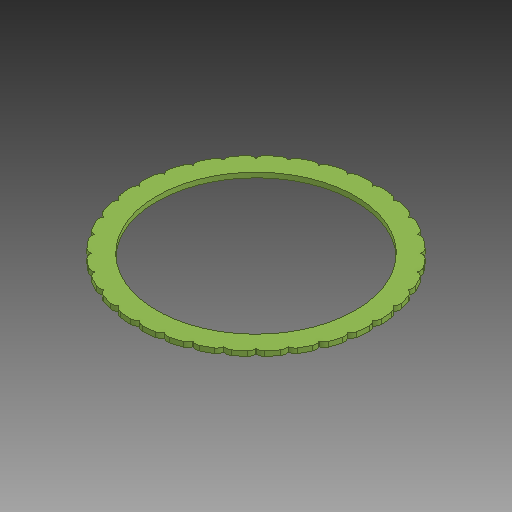
# Autodesk Inventor part: tsop_board
Saved by Autodesk Inventor 2020 (Build 240168000, 168)
## iProperties
Created: 2024-11-04
Part Number: tsop_board
Material: Медь
Document SubType Name: Modeling
Designer: Ivan
Density: 8.94 g/cm^3
Appearance: Оливково-зеленый
Mass: 41.749 g
Surface Area: 58.5361 cm^2
Volume: 4.66991 cm^3
Author: Ivan
Autodesk Inventor part; units mm, degrees
ref_plane "YZ Plane" through (0, 0, 0) normal (1, 0, 0) x (0, 1, 0)
ref_plane "XZ Plane" through (0, 0, 0) normal (0, 1, 0) x (-1, 0, 0)
ref_plane "XY Plane" through (0, 0, 0) normal (0, 0, 1) x (1, 0, 0)
sketch "Эскиз1" plane through (0, 0, 0) normal (0, 1, 0) x (-1, 0, 0)
  line L0 (48.1278, 3.6) -> (42.9278, 3.6)
  line L1 (42.9278, 3.6) -> (42.9278, -3.6)
  line L2 (42.9278, -3.6) -> (48.1278, -3.6)
  line L3 (48.1278, -3.6) -> (48.1278, 3.6)
  line L4 (0, 0) -> (42.9278, 0) construction
  circle A0 centre (0, 0) radius 45.67 construction
  line L5 (45.5278, 3.6) -> (45.5278, -3.6) construction
  line L6 (41.4007, 11.9056) -> (42.8053, 4.844)
  line L7 (46.5008, 12.9201) -> (41.4007, 11.9056)
  line L8 (47.9054, 5.8585) -> (46.5008, 12.9201)
  line L9 (42.8053, 4.844) -> (47.9054, 5.8585)
  line L10 (38.2825, 19.7537) -> (41.0378, 13.1018)
  line L11 (43.0867, 21.7437) -> (38.2825, 19.7537)
  line L12 (45.842, 15.0918) -> (43.0867, 21.7437)
  line L13 (41.0378, 13.1018) -> (45.842, 15.0918)
  line L14 (33.6931, 26.8427) -> (37.6933, 20.8561)
  line L15 (38.0168, 29.7317) -> (33.6931, 26.8427)
  line L16 (42.0169, 23.7451) -> (38.0168, 29.7317)
  line L17 (37.6933, 20.8561) -> (42.0169, 23.7451)
  line L18 (27.809, 32.9002) -> (32.9002, 27.809)
  line L19 (31.4859, 36.5771) -> (27.809, 32.9002)
  line L20 (36.5771, 31.4859) -> (31.4859, 36.5771)
  line L21 (32.9002, 27.809) -> (36.5771, 31.4859)
  line L22 (20.8561, 37.6933) -> (26.8427, 33.6931)
  line L23 (23.7451, 42.0169) -> (20.8561, 37.6933)
  line L24 (29.7317, 38.0168) -> (23.7451, 42.0169)
  line L25 (26.8427, 33.6931) -> (29.7317, 38.0168)
  line L26 (13.1018, 41.0378) -> (19.7537, 38.2825)
  line L27 (15.0918, 45.842) -> (13.1018, 41.0378)
  line L28 (21.7437, 43.0867) -> (15.0918, 45.842)
  line L29 (19.7537, 38.2825) -> (21.7437, 43.0867)
  line L30 (4.844, 42.8053) -> (11.9056, 41.4007)
  line L31 (5.8585, 47.9054) -> (4.844, 42.8053)
  line L32 (12.9201, 46.5008) -> (5.8585, 47.9054)
  line L33 (11.9056, 41.4007) -> (12.9201, 46.5008)
  line L34 (-3.6, 42.9278) -> (3.6, 42.9278)
  line L35 (-3.6, 48.1278) -> (-3.6, 42.9278)
  line L36 (3.6, 48.1278) -> (-3.6, 48.1278)
  line L37 (3.6, 42.9278) -> (3.6, 48.1278)
  line L38 (-11.9056, 41.4007) -> (-4.844, 42.8053)
  line L39 (-12.9201, 46.5008) -> (-11.9056, 41.4007)
  line L40 (-5.8585, 47.9054) -> (-12.9201, 46.5008)
  line L41 (-4.844, 42.8053) -> (-5.8585, 47.9054)
  line L42 (-19.7537, 38.2825) -> (-13.1018, 41.0378)
  line L43 (-21.7437, 43.0867) -> (-19.7537, 38.2825)
  line L44 (-15.0918, 45.842) -> (-21.7437, 43.0867)
  line L45 (-13.1018, 41.0378) -> (-15.0918, 45.842)
  line L46 (-26.8427, 33.6931) -> (-20.8561, 37.6933)
  line L47 (-29.7317, 38.0168) -> (-26.8427, 33.6931)
  line L48 (-23.7451, 42.0169) -> (-29.7317, 38.0168)
  line L49 (-20.8561, 37.6933) -> (-23.7451, 42.0169)
  line L50 (-32.9002, 27.809) -> (-27.809, 32.9002)
  line L51 (-36.5771, 31.4859) -> (-32.9002, 27.809)
  line L52 (-31.4859, 36.5771) -> (-36.5771, 31.4859)
  line L53 (-27.809, 32.9002) -> (-31.4859, 36.5771)
  line L54 (-37.6933, 20.8561) -> (-33.6931, 26.8427)
  line L55 (-42.0169, 23.7451) -> (-37.6933, 20.8561)
  line L56 (-38.0168, 29.7317) -> (-42.0169, 23.7451)
  line L57 (-33.6931, 26.8427) -> (-38.0168, 29.7317)
  line L58 (-41.0378, 13.1018) -> (-38.2825, 19.7537)
  line L59 (-45.842, 15.0918) -> (-41.0378, 13.1018)
  line L60 (-43.0867, 21.7437) -> (-45.842, 15.0918)
  line L61 (-38.2825, 19.7537) -> (-43.0867, 21.7437)
  line L62 (-42.8053, 4.844) -> (-41.4007, 11.9056)
  line L63 (-47.9054, 5.8585) -> (-42.8053, 4.844)
  line L64 (-46.5008, 12.9201) -> (-47.9054, 5.8585)
  line L65 (-41.4007, 11.9056) -> (-46.5008, 12.9201)
  line L66 (-42.9278, -3.6) -> (-42.9278, 3.6)
  line L67 (-48.1278, -3.6) -> (-42.9278, -3.6)
  line L68 (-48.1278, 3.6) -> (-48.1278, -3.6)
  line L69 (-42.9278, 3.6) -> (-48.1278, 3.6)
  line L70 (-41.4007, -11.9056) -> (-42.8053, -4.844)
  line L71 (-46.5008, -12.9201) -> (-41.4007, -11.9056)
  line L72 (-47.9054, -5.8585) -> (-46.5008, -12.9201)
  line L73 (-42.8053, -4.844) -> (-47.9054, -5.8585)
  line L74 (-38.2825, -19.7537) -> (-41.0378, -13.1018)
  line L75 (-43.0867, -21.7437) -> (-38.2825, -19.7537)
  line L76 (-45.842, -15.0918) -> (-43.0867, -21.7437)
  line L77 (-41.0378, -13.1018) -> (-45.842, -15.0918)
  line L78 (-33.6931, -26.8427) -> (-37.6933, -20.8561)
  line L79 (-38.0168, -29.7317) -> (-33.6931, -26.8427)
  line L80 (-42.0169, -23.7451) -> (-38.0168, -29.7317)
  line L81 (-37.6933, -20.8561) -> (-42.0169, -23.7451)
  line L82 (-27.809, -32.9002) -> (-32.9002, -27.809)
  line L83 (-31.4859, -36.5771) -> (-27.809, -32.9002)
  line L84 (-36.5771, -31.4859) -> (-31.4859, -36.5771)
  line L85 (-32.9002, -27.809) -> (-36.5771, -31.4859)
  line L86 (-20.8561, -37.6933) -> (-26.8427, -33.6931)
  line L87 (-23.7451, -42.0169) -> (-20.8561, -37.6933)
  line L88 (-29.7317, -38.0168) -> (-23.7451, -42.0169)
  line L89 (-26.8427, -33.6931) -> (-29.7317, -38.0168)
  line L90 (-13.1018, -41.0378) -> (-19.7537, -38.2825)
  line L91 (-15.0918, -45.842) -> (-13.1018, -41.0378)
  line L92 (-21.7437, -43.0867) -> (-15.0918, -45.842)
  line L93 (-19.7537, -38.2825) -> (-21.7437, -43.0867)
  line L94 (-4.844, -42.8053) -> (-11.9056, -41.4007)
  line L95 (-5.8585, -47.9054) -> (-4.844, -42.8053)
  line L96 (-12.9201, -46.5008) -> (-5.8585, -47.9054)
  line L97 (-11.9056, -41.4007) -> (-12.9201, -46.5008)
  line L98 (3.6, -42.9278) -> (-3.6, -42.9278)
  line L99 (3.6, -48.1278) -> (3.6, -42.9278)
  line L100 (-3.6, -48.1278) -> (3.6, -48.1278)
  line L101 (-3.6, -42.9278) -> (-3.6, -48.1278)
  line L102 (11.9056, -41.4007) -> (4.844, -42.8053)
  line L103 (12.9201, -46.5008) -> (11.9056, -41.4007)
  line L104 (5.8585, -47.9054) -> (12.9201, -46.5008)
  line L105 (4.844, -42.8053) -> (5.8585, -47.9054)
  line L106 (19.7537, -38.2825) -> (13.1018, -41.0378)
  line L107 (21.7437, -43.0867) -> (19.7537, -38.2825)
  line L108 (15.0918, -45.842) -> (21.7437, -43.0867)
  line L109 (13.1018, -41.0378) -> (15.0918, -45.842)
  line L110 (26.8427, -33.6931) -> (20.8561, -37.6933)
  line L111 (29.7317, -38.0168) -> (26.8427, -33.6931)
  line L112 (23.7451, -42.0169) -> (29.7317, -38.0168)
  line L113 (20.8561, -37.6933) -> (23.7451, -42.0169)
  line L114 (32.9002, -27.809) -> (27.809, -32.9002)
  line L115 (36.5771, -31.4859) -> (32.9002, -27.809)
  line L116 (31.4859, -36.5771) -> (36.5771, -31.4859)
  line L117 (27.809, -32.9002) -> (31.4859, -36.5771)
  line L118 (37.6933, -20.8561) -> (33.6931, -26.8427)
  line L119 (42.0169, -23.7451) -> (37.6933, -20.8561)
  line L120 (38.0168, -29.7317) -> (42.0169, -23.7451)
  line L121 (33.6931, -26.8427) -> (38.0168, -29.7317)
  line L122 (41.0378, -13.1018) -> (38.2825, -19.7537)
  line L123 (45.842, -15.0918) -> (41.0378, -13.1018)
  line L124 (43.0867, -21.7437) -> (45.842, -15.0918)
  line L125 (38.2825, -19.7537) -> (43.0867, -21.7437)
  line L126 (42.8053, -4.844) -> (41.4007, -11.9056)
  line L127 (47.9054, -5.8585) -> (42.8053, -4.844)
  line L128 (46.5008, -12.9201) -> (47.9054, -5.8585)
  line L129 (41.4007, -11.9056) -> (46.5008, -12.9201)
  line L130 (42.8053, 4.844) -> (42.9278, 3.6) construction
  line L131 (42.9278, 3.6) -> (46.884, 3.9896) construction
  point P0 (45.67, 0)
  point P1 (42.103, 8.3748)
  point P2 (43.9507, 12.4129)
  point P3 (45.3554, 5.3512)
  point P4 (39.6602, 16.4278)
  point P5 (40.6846, 20.7487)
  point P6 (43.4399, 14.0968)
  point P7 (35.6932, 23.8494)
  point P8 (35.855, 28.2872)
  point P9 (39.8551, 22.3006)
  point P10 (30.3546, 30.3546)
  point P11 (29.6475, 34.7386)
  point P12 (34.7386, 29.6475)
  point P13 (23.8494, 35.6932)
  point P14 (22.3006, 39.8551)
  point P15 (28.2872, 35.855)
  point P16 (16.4278, 39.6602)
  point P17 (14.0968, 43.4399)
  point P18 (20.7487, 40.6846)
  point P19 (8.3748, 42.103)
  point P20 (5.3512, 45.3554)
  point P21 (12.4129, 43.9507)
  point P22 (0, 42.9278)
  point P23 (-3.6, 45.5278)
  point P24 (3.6, 45.5278)
  point P25 (-8.3748, 42.103)
  point P26 (-12.4129, 43.9507)
  point P27 (-5.3512, 45.3554)
  point P28 (-16.4278, 39.6602)
  point P29 (-20.7487, 40.6846)
  point P30 (-14.0968, 43.4399)
  point P31 (-23.8494, 35.6932)
  point P32 (-28.2872, 35.855)
  point P33 (-22.3006, 39.8551)
  point P34 (-30.3546, 30.3546)
  point P35 (-34.7386, 29.6475)
  point P36 (-29.6475, 34.7386)
  point P37 (-35.6932, 23.8494)
  point P38 (-39.8551, 22.3006)
  point P39 (-35.855, 28.2872)
  point P40 (-39.6602, 16.4278)
  point P41 (-43.4399, 14.0968)
  point P42 (-40.6846, 20.7487)
  point P43 (-42.103, 8.3748)
  point P44 (-45.3554, 5.3512)
  point P45 (-43.9507, 12.4129)
  point P46 (-42.9278, 0)
  point P47 (-45.5278, -3.6)
  point P48 (-45.5278, 3.6)
  point P49 (-42.103, -8.3748)
  point P50 (-43.9507, -12.4129)
  point P51 (-45.3554, -5.3512)
  point P52 (-39.6602, -16.4278)
  point P53 (-40.6846, -20.7487)
  point P54 (-43.4399, -14.0968)
  point P55 (-35.6932, -23.8494)
  point P56 (-35.855, -28.2872)
  point P57 (-39.8551, -22.3006)
  point P58 (-30.3546, -30.3546)
  point P59 (-29.6475, -34.7386)
  point P60 (-34.7386, -29.6475)
  point P61 (-23.8494, -35.6932)
  point P62 (-22.3006, -39.8551)
  point P63 (-28.2872, -35.855)
  point P64 (-16.4278, -39.6602)
  point P65 (-14.0968, -43.4399)
  point P66 (-20.7487, -40.6846)
  point P67 (-8.3748, -42.103)
  point P68 (-5.3512, -45.3554)
  point P69 (-12.4129, -43.9507)
  point P70 (0, -42.9278)
  point P71 (3.6, -45.5278)
  point P72 (-3.6, -45.5278)
  point P73 (8.3748, -42.103)
  point P74 (12.4129, -43.9507)
  point P75 (5.3512, -45.3554)
  point P76 (16.4278, -39.6602)
  point P77 (20.7487, -40.6846)
  point P78 (14.0968, -43.4399)
  point P79 (23.8494, -35.6932)
  point P80 (28.2872, -35.855)
  point P81 (22.3006, -39.8551)
  point P82 (30.3546, -30.3546)
  point P83 (34.7386, -29.6475)
  point P84 (29.6475, -34.7386)
  point P85 (35.6932, -23.8494)
  point P86 (39.8551, -22.3006)
  point P87 (35.855, -28.2872)
  point P88 (39.6602, -16.4278)
  point P89 (43.4399, -14.0968)
  point P90 (40.6846, -20.7487)
  point P91 (42.103, -8.3748)
  point P92 (45.3554, -5.3512)
  point P93 (43.9507, -12.4129)
sketch "Эскиз3" plane through (0, 0, 0) normal (0, 1, 0) x (-1, 0, 0)
  line L0 (42.8053, 4.844) -> (42.9278, 3.6) construction
  line L1 (42.8666, 4.222) -> (50.4728, 4.9711) construction
  line L2 (48.1278, -3.6) -> (48.1278, 3.6)
  line L3 (48.1278, -0.05) -> (48.1278, 0.05)
  line L4 (48.1278, 2.45) -> (49.3278, 2.45) construction
  arc A0 (48.1278, 0.05) -> (49.3278, 2.45) centre (46.3278, 2.45) ccw
  line L5 (49.3278, 2.45) -> (49.3278, 0) construction
  line L6 (0, 0) -> (42.9278, 0) construction
  arc A1 (49.3278, -2.45) -> (48.1278, -0.05) centre (46.3278, -2.45) ccw
  arc A2 (47.1933, 9.4383) -> (47.9021, 12.0263) centre (44.9597, 11.441) ccw
  arc A3 (48.858, 7.2205) -> (47.2128, 9.3402) centre (45.9156, 6.6352) ccw
  line L7 (47.2128, 9.3402) -> (47.1933, 9.4383)
  arc A4 (44.4452, 18.4639) -> (44.6354, 21.1405) centre (41.8638, 19.9924) ccw
  arc A5 (46.5106, 16.6134) -> (44.4835, 18.3715) centre (43.7389, 15.4654) ccw
  line L8 (44.4835, 18.3715) -> (44.4452, 18.4639)
  arc A6 (39.9891, 26.78) -> (39.6535, 29.4422) centre (37.1591, 27.7755) ccw
  arc A7 (42.3758, 25.368) -> (40.0446, 26.6968) centre (39.8813, 23.7013) ccw
  line L9 (40.0446, 26.6968) -> (39.9891, 26.78)
  arc A8 (33.9962, 34.0669) -> (33.1476, 36.6125) centre (31.0263, 34.4911) ccw
  arc A9 (36.6125, 33.1476) -> (34.0669, 33.9962) centre (34.4911, 31.0263) ccw
  line L10 (34.0669, 33.9962) -> (33.9962, 34.0669)
  arc A10 (26.6968, 40.0446) -> (25.368, 42.3758) centre (23.7013, 39.8813) ccw
  arc A11 (29.4422, 39.6535) -> (26.78, 39.9891) centre (27.7755, 37.1591) ccw
  line L11 (26.78, 39.9891) -> (26.6968, 40.0446)
  arc A12 (18.3715, 44.4835) -> (16.6134, 46.5106) centre (15.4654, 43.7389) ccw
  arc A13 (21.1405, 44.6354) -> (18.4639, 44.4452) centre (19.9924, 41.8638) ccw
  line L12 (18.4639, 44.4452) -> (18.3715, 44.4835)
  arc A14 (9.3402, 47.2128) -> (7.2205, 48.858) centre (6.6352, 45.9156) ccw
  arc A15 (12.0263, 47.9021) -> (9.4383, 47.1933) centre (11.441, 44.9597) ccw
  line L13 (9.4383, 47.1933) -> (9.3402, 47.2128)
  arc A16 (-0.05, 48.1278) -> (-2.45, 49.3278) centre (-2.45, 46.3278) ccw
  arc A17 (2.45, 49.3278) -> (0.05, 48.1278) centre (2.45, 46.3278) ccw
  line L14 (0.05, 48.1278) -> (-0.05, 48.1278)
  arc A18 (-9.4383, 47.1933) -> (-12.0263, 47.9021) centre (-11.441, 44.9597) ccw
  arc A19 (-7.2205, 48.858) -> (-9.3402, 47.2128) centre (-6.6352, 45.9156) ccw
  line L15 (-9.3402, 47.2128) -> (-9.4383, 47.1933)
  arc A20 (-18.4639, 44.4452) -> (-21.1405, 44.6354) centre (-19.9924, 41.8638) ccw
  arc A21 (-16.6134, 46.5106) -> (-18.3715, 44.4835) centre (-15.4654, 43.7389) ccw
  line L16 (-18.3715, 44.4835) -> (-18.4639, 44.4452)
  arc A22 (-26.78, 39.9891) -> (-29.4422, 39.6535) centre (-27.7755, 37.1591) ccw
  arc A23 (-25.368, 42.3758) -> (-26.6968, 40.0446) centre (-23.7013, 39.8813) ccw
  line L17 (-26.6968, 40.0446) -> (-26.78, 39.9891)
  arc A24 (-34.0669, 33.9962) -> (-36.6125, 33.1476) centre (-34.4911, 31.0263) ccw
  arc A25 (-33.1476, 36.6125) -> (-33.9962, 34.0669) centre (-31.0263, 34.4911) ccw
  line L18 (-33.9962, 34.0669) -> (-34.0669, 33.9962)
  arc A26 (-40.0446, 26.6968) -> (-42.3758, 25.368) centre (-39.8813, 23.7013) ccw
  arc A27 (-39.6535, 29.4422) -> (-39.9891, 26.78) centre (-37.1591, 27.7755) ccw
  line L19 (-39.9891, 26.78) -> (-40.0446, 26.6968)
  arc A28 (-44.4835, 18.3715) -> (-46.5106, 16.6134) centre (-43.7389, 15.4654) ccw
  arc A29 (-44.6354, 21.1405) -> (-44.4452, 18.4639) centre (-41.8638, 19.9924) ccw
  line L20 (-44.4452, 18.4639) -> (-44.4835, 18.3715)
  arc A30 (-47.2128, 9.3402) -> (-48.858, 7.2205) centre (-45.9156, 6.6352) ccw
  arc A31 (-47.9021, 12.0263) -> (-47.1933, 9.4383) centre (-44.9597, 11.441) ccw
  line L21 (-47.1933, 9.4383) -> (-47.2128, 9.3402)
  arc A32 (-48.1278, -0.05) -> (-49.3278, -2.45) centre (-46.3278, -2.45) ccw
  arc A33 (-49.3278, 2.45) -> (-48.1278, 0.05) centre (-46.3278, 2.45) ccw
  line L22 (-48.1278, 0.05) -> (-48.1278, -0.05)
  arc A34 (-47.1933, -9.4383) -> (-47.9021, -12.0263) centre (-44.9597, -11.441) ccw
  arc A35 (-48.858, -7.2205) -> (-47.2128, -9.3402) centre (-45.9156, -6.6352) ccw
  line L23 (-47.2128, -9.3402) -> (-47.1933, -9.4383)
  arc A36 (-44.4452, -18.4639) -> (-44.6354, -21.1405) centre (-41.8638, -19.9924) ccw
  arc A37 (-46.5106, -16.6134) -> (-44.4835, -18.3715) centre (-43.7389, -15.4654) ccw
  line L24 (-44.4835, -18.3715) -> (-44.4452, -18.4639)
  arc A38 (-39.9891, -26.78) -> (-39.6535, -29.4422) centre (-37.1591, -27.7755) ccw
  arc A39 (-42.3758, -25.368) -> (-40.0446, -26.6968) centre (-39.8813, -23.7013) ccw
  line L25 (-40.0446, -26.6968) -> (-39.9891, -26.78)
  arc A40 (-33.9962, -34.0669) -> (-33.1476, -36.6125) centre (-31.0263, -34.4911) ccw
  arc A41 (-36.6125, -33.1476) -> (-34.0669, -33.9962) centre (-34.4911, -31.0263) ccw
  line L26 (-34.0669, -33.9962) -> (-33.9962, -34.0669)
  arc A42 (-26.6968, -40.0446) -> (-25.368, -42.3758) centre (-23.7013, -39.8813) ccw
  arc A43 (-29.4422, -39.6535) -> (-26.78, -39.9891) centre (-27.7755, -37.1591) ccw
  line L27 (-26.78, -39.9891) -> (-26.6968, -40.0446)
  arc A44 (-18.3715, -44.4835) -> (-16.6134, -46.5106) centre (-15.4654, -43.7389) ccw
  arc A45 (-21.1405, -44.6354) -> (-18.4639, -44.4452) centre (-19.9924, -41.8638) ccw
  line L28 (-18.4639, -44.4452) -> (-18.3715, -44.4835)
  arc A46 (-9.3402, -47.2128) -> (-7.2205, -48.858) centre (-6.6352, -45.9156) ccw
  arc A47 (-12.0263, -47.9021) -> (-9.4383, -47.1933) centre (-11.441, -44.9597) ccw
  line L29 (-9.4383, -47.1933) -> (-9.3402, -47.2128)
  arc A48 (0.05, -48.1278) -> (2.45, -49.3278) centre (2.45, -46.3278) ccw
  arc A49 (-2.45, -49.3278) -> (-0.05, -48.1278) centre (-2.45, -46.3278) ccw
  line L30 (-0.05, -48.1278) -> (0.05, -48.1278)
  arc A50 (9.4383, -47.1933) -> (12.0263, -47.9021) centre (11.441, -44.9597) ccw
  arc A51 (7.2205, -48.858) -> (9.3402, -47.2128) centre (6.6352, -45.9156) ccw
  line L31 (9.3402, -47.2128) -> (9.4383, -47.1933)
  arc A52 (18.4639, -44.4452) -> (21.1405, -44.6354) centre (19.9924, -41.8638) ccw
  arc A53 (16.6134, -46.5106) -> (18.3715, -44.4835) centre (15.4654, -43.7389) ccw
  line L32 (18.3715, -44.4835) -> (18.4639, -44.4452)
  arc A54 (26.78, -39.9891) -> (29.4422, -39.6535) centre (27.7755, -37.1591) ccw
  arc A55 (25.368, -42.3758) -> (26.6968, -40.0446) centre (23.7013, -39.8813) ccw
  line L33 (26.6968, -40.0446) -> (26.78, -39.9891)
  arc A56 (34.0669, -33.9962) -> (36.6125, -33.1476) centre (34.4911, -31.0263) ccw
  arc A57 (33.1476, -36.6125) -> (33.9962, -34.0669) centre (31.0263, -34.4911) ccw
  line L34 (33.9962, -34.0669) -> (34.0669, -33.9962)
  arc A58 (40.0446, -26.6968) -> (42.3758, -25.368) centre (39.8813, -23.7013) ccw
  arc A59 (39.6535, -29.4422) -> (39.9891, -26.78) centre (37.1591, -27.7755) ccw
  line L35 (39.9891, -26.78) -> (40.0446, -26.6968)
  arc A60 (44.4835, -18.3715) -> (46.5106, -16.6134) centre (43.7389, -15.4654) ccw
  arc A61 (44.6354, -21.1405) -> (44.4452, -18.4639) centre (41.8638, -19.9924) ccw
  line L36 (44.4452, -18.4639) -> (44.4835, -18.3715)
  arc A62 (47.2128, -9.3402) -> (48.858, -7.2205) centre (45.9156, -6.6352) ccw
  arc A63 (47.9021, -12.0263) -> (47.1933, -9.4383) centre (44.9597, -11.441) ccw
  line L37 (47.1933, -9.4383) -> (47.2128, -9.3402)
  arc A64 (49.3278, 2.45) -> (48.858, 7.2205) centre (0, 0) ccw
  arc A65 (47.9021, 12.0263) -> (46.5106, 16.6134) centre (0, 0) ccw
  arc A66 (44.6354, 21.1405) -> (42.3758, 25.368) centre (0, 0) ccw
  arc A67 (39.6535, 29.4422) -> (36.6125, 33.1476) centre (0, 0) ccw
  arc A68 (33.1476, 36.6125) -> (29.4422, 39.6535) centre (0, 0) ccw
  arc A69 (25.368, 42.3758) -> (21.1405, 44.6354) centre (0, 0) ccw
  arc A70 (16.6134, 46.5106) -> (12.0263, 47.9021) centre (0, 0) ccw
  arc A71 (7.2205, 48.858) -> (2.45, 49.3278) centre (0, 0) ccw
  arc A72 (-2.45, 49.3278) -> (-7.2205, 48.858) centre (0, 0) ccw
  arc A73 (-12.0263, 47.9021) -> (-16.6134, 46.5106) centre (0, 0) ccw
  arc A74 (-21.1405, 44.6354) -> (-25.368, 42.3758) centre (0, 0) ccw
  arc A75 (-29.4422, 39.6535) -> (-33.1476, 36.6125) centre (0, 0) ccw
  arc A76 (-36.6125, 33.1476) -> (-39.6535, 29.4422) centre (0, 0) ccw
  arc A77 (-42.3758, 25.368) -> (-44.6354, 21.1405) centre (0, 0) ccw
  arc A78 (-46.5106, 16.6134) -> (-47.9021, 12.0263) centre (0, 0) ccw
  arc A79 (-48.858, 7.2205) -> (-49.3278, 2.45) centre (0, 0) ccw
  arc A80 (-49.3278, -2.45) -> (-48.858, -7.2205) centre (0, 0) ccw
  arc A81 (-47.9021, -12.0263) -> (-46.5106, -16.6134) centre (0, 0) ccw
  arc A82 (-44.6354, -21.1405) -> (-42.3758, -25.368) centre (0, 0) ccw
  arc A83 (-39.6535, -29.4422) -> (-36.6125, -33.1476) centre (0, 0) ccw
  arc A84 (-33.1476, -36.6125) -> (-29.4422, -39.6535) centre (0, 0) ccw
  arc A85 (-25.368, -42.3758) -> (-21.1405, -44.6354) centre (0, 0) ccw
  arc A86 (-16.6134, -46.5106) -> (-12.0263, -47.9021) centre (0, 0) ccw
  arc A87 (-7.2205, -48.858) -> (-2.45, -49.3278) centre (0, 0) ccw
  arc A88 (2.45, -49.3278) -> (7.2205, -48.858) centre (0, 0) ccw
  arc A89 (12.0263, -47.9021) -> (16.6134, -46.5106) centre (0, 0) ccw
  arc A90 (21.1405, -44.6354) -> (25.368, -42.3758) centre (0, 0) ccw
  arc A91 (29.4422, -39.6535) -> (33.1476, -36.6125) centre (0, 0) ccw
  arc A92 (36.6125, -33.1476) -> (39.6535, -29.4422) centre (0, 0) ccw
  arc A93 (42.3758, -25.368) -> (44.6354, -21.1405) centre (0, 0) ccw
  arc A94 (46.5106, -16.6134) -> (47.9021, -12.0263) centre (0, 0) ccw
  arc A95 (48.858, -7.2205) -> (49.3278, -2.45) centre (0, 0) ccw
  circle A96 centre (0, 0) radius 40.9278
  line L38 (42.9278, 3.6) -> (42.9278, -3.6)
  point P0 (48.1278, 0)
  point P1 (47.2031, 9.3893)
  point P2 (44.4643, 18.4177)
  point P3 (40.0168, 26.7384)
  point P4 (34.0315, 34.0315)
  point P5 (26.7384, 40.0168)
  point P6 (18.4177, 44.4643)
  point P7 (9.3893, 47.2031)
  point P8 (0, 48.1278)
  point P9 (-9.3893, 47.2031)
  point P10 (-18.4177, 44.4643)
  point P11 (-26.7384, 40.0168)
  point P12 (-34.0315, 34.0315)
  point P13 (-40.0168, 26.7384)
  point P14 (-44.4643, 18.4177)
  point P15 (-47.2031, 9.3893)
  point P16 (-48.1278, 0)
  point P17 (-47.2031, -9.3893)
  point P18 (-44.4643, -18.4177)
  point P19 (-40.0168, -26.7384)
  point P20 (-34.0315, -34.0315)
  point P21 (-26.7384, -40.0168)
  point P22 (-18.4177, -44.4643)
  point P23 (-9.3893, -47.2031)
  point P24 (0, -48.1278)
  point P25 (9.3893, -47.2031)
  point P26 (18.4177, -44.4643)
  point P27 (26.7384, -40.0168)
  point P28 (34.0315, -34.0315)
  point P29 (40.0168, -26.7384)
  point P30 (44.4643, -18.4177)
  point P31 (47.2031, -9.3893)
  point P32 (40.9278, 0)
  point P33 (48.858, -7.2205)
  point P34 (49.3278, -2.45)
  point P35 (48.1278, -0.05)
  point P36 (48.1278, 0.05)
  point P37 (47.9021, 12.0263)
  point P38 (46.5106, 16.6134)
  point P39 (44.6354, 21.1405)
  point P40 (42.3758, 25.368)
  point P41 (39.6535, 29.4422)
  point P42 (36.6125, 33.1476)
  point P43 (33.1476, 36.6125)
  point P44 (29.4422, 39.6535)
  point P45 (25.368, 42.3758)
  point P46 (21.1405, 44.6354)
  point P47 (16.6134, 46.5106)
  point P48 (12.0263, 47.9021)
  point P49 (7.2205, 48.858)
  point P50 (2.45, 49.3278)
  point P51 (-2.45, 49.3278)
  point P52 (-7.2205, 48.858)
  point P53 (-12.0263, 47.9021)
  point P54 (-16.6134, 46.5106)
  point P55 (-21.1405, 44.6354)
  point P56 (-25.368, 42.3758)
  point P57 (-29.4422, 39.6535)
  point P58 (-33.1476, 36.6125)
  point P59 (-36.6125, 33.1476)
  point P60 (-39.6535, 29.4422)
  point P61 (-42.3758, 25.368)
  point P62 (-44.6354, 21.1405)
  point P63 (-46.5106, 16.6134)
  point P64 (-47.9021, 12.0263)
  point P65 (-48.858, 7.2205)
  point P66 (-49.3278, 2.45)
  point P67 (-49.3278, -2.45)
  point P68 (-48.858, -7.2205)
  point P69 (-47.9021, -12.0263)
  point P70 (-46.5106, -16.6134)
  point P71 (-44.6354, -21.1405)
  point P72 (-42.3758, -25.368)
  point P73 (-39.6535, -29.4422)
  point P74 (-36.6125, -33.1476)
  point P75 (-33.1476, -36.6125)
  point P76 (-29.4422, -39.6535)
  point P77 (-25.368, -42.3758)
  point P78 (-21.1405, -44.6354)
  point P79 (-16.6134, -46.5106)
  point P80 (-12.0263, -47.9021)
  point P81 (-7.2205, -48.858)
  point P82 (-2.45, -49.3278)
  point P83 (2.45, -49.3278)
  point P84 (7.2205, -48.858)
  point P85 (12.0263, -47.9021)
  point P86 (16.6134, -46.5106)
  point P87 (21.1405, -44.6354)
  point P88 (25.368, -42.3758)
  point P89 (29.4422, -39.6535)
  point P90 (33.1476, -36.6125)
  point P91 (36.6125, -33.1476)
  point P92 (39.6535, -29.4422)
  point P93 (42.3758, -25.368)
  point P94 (44.6354, -21.1405)
  point P95 (46.5106, -16.6134)
  point P96 (47.9021, -12.0263)
extrude "Выдавливание1" add sketch "Эскиз3" along normal blind 2
